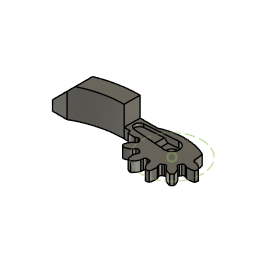
TRGRIP01_Grip_Right_50x15 (Autodesk Fusion 360 design; units mm, degrees)
description: Spur Gear; Module: 2.5; Num Teeth: 12; Pressure Angle: 20.0; Backlash: 0.00 mm
Autodesk Fusion 360 part; units mm, degrees
sketch "스케치1" plane through (0, 0, 0) normal (0, 0, 1) x (1, 0, 0) in component "Spur Gear (12 teeth)"
  circle A0 centre (0, 0) radius 11.9492
  circle A1 centre (0, 0) radius 2.5
sketch "스케치2" plane through (0, 0, 0) normal (0, 0, 1) x (1, 0, 0) in component "Spur Gear (12 teeth)"
  spline S0 degree 5 poles (13.9458, -2.0479) (13.9559, -2.0494) (13.9759, -2.052) (14.0061, -2.0549) (14.0465, -2.057) (14.0972, -2.0572) (14.1481, -2.0556) (14.199, -2.0528) (14.2501, -2.0495) (14.3011, -2.0457) (14.3522, -2.0415) (14.4034, -2.0367) (14.4546, -2.0311) (14.5058, -2.0247) (14.5571, -2.0173) (14.6084, -2.0091) (14.6597, -2.0003) (14.7111, -1.9908) (14.7624, -1.9808) (14.8137, -1.9703) (14.8651, -1.9594) (14.9164, -1.9479) (14.9678, -1.9358) (15.0191, -1.9232) (15.0705, -1.91) (15.1218, -1.8963) (15.1731, -1.882) (15.2244, -1.8673) (15.2757, -1.8521) (15.3269, -1.8365) (15.3781, -1.8204) (15.4293, -1.8038) (15.4805, -1.7868) (15.5316, -1.7693) (15.5827, -1.7513) (15.6338, -1.7329) (15.6848, -1.7141) (15.7358, -1.6948) (15.7868, -1.6751) (15.8377, -1.655) (15.8886, -1.6345) (15.9394, -1.6136) (15.9902, -1.5922) (16.0409, -1.5705) (16.0916, -1.5483) (16.1422, -1.5258) (16.1928, -1.5028) (16.2433, -1.4794) (16.2937, -1.4557) (16.3441, -1.4316) (16.3944, -1.4071) (16.4447, -1.3822) (16.4949, -1.3569) (16.545, -1.3313) (16.5951, -1.3053) (16.6451, -1.2789) (16.695, -1.2521) (16.7448, -1.225) (16.7946, -1.1975) (16.8443, -1.1697) (16.8939, -1.1415) (16.9435, -1.1129) (16.9929, -1.084) (17.0423, -1.0548) (17.0916, -1.0251) (17.1408, -0.9952) (17.1899, -0.9649) (17.239, -0.9343) (17.2879, -0.9033) (17.3368, -0.8719) (17.3856, -0.8403) (17.4245, -0.8147) (17.4537, -0.7953) (17.4731, -0.7824) (17.4828, -0.7759) knots 0 0 0 0 0 0 0.01428571 0.02857143 0.04285714 0.05714286 0.07142857 0.08571429 0.1 0.11428571 0.12857143 0.14285714 0.15714286 0.17142857 0.18571429 0.2 0.21428571 0.22857143 0.24285714 0.25714286 0.27142857 0.28571429 0.3 0.31428571 0.32857143 0.34285714 0.35714286 0.37142857 0.38571429 0.4 0.41428571 0.42857143 0.44285714 0.45714286 0.47142857 0.48571429 0.5 0.51428571 0.52857143 0.54285714 0.55714286 0.57142857 0.58571429 0.6 0.61428571 0.62857143 0.64285714 0.65714286 0.67142857 0.68571429 0.7 0.71428571 0.72857143 0.74285714 0.75714286 0.77142857 0.78571429 0.8 0.81428571 0.82857143 0.84285714 0.85714286 0.87142857 0.88571429 0.9 0.91428571 0.92857143 0.94285714 0.95714286 0.97142857 0.98571429 1 1 1 1 1 1
  spline S1 degree 5 poles (13.9458, 2.0479) (13.9559, 2.0494) (13.9759, 2.052) (14.0061, 2.0549) (14.0465, 2.057) (14.0972, 2.0572) (14.1481, 2.0556) (14.199, 2.0528) (14.2501, 2.0495) (14.3011, 2.0457) (14.3522, 2.0415) (14.4034, 2.0367) (14.4546, 2.0311) (14.5058, 2.0247) (14.5571, 2.0173) (14.6084, 2.0091) (14.6597, 2.0003) (14.7111, 1.9908) (14.7624, 1.9808) (14.8137, 1.9703) (14.8651, 1.9594) (14.9164, 1.9479) (14.9678, 1.9358) (15.0191, 1.9232) (15.0705, 1.91) (15.1218, 1.8963) (15.1731, 1.882) (15.2244, 1.8673) (15.2757, 1.8521) (15.3269, 1.8365) (15.3781, 1.8204) (15.4293, 1.8038) (15.4805, 1.7868) (15.5316, 1.7693) (15.5827, 1.7513) (15.6338, 1.7329) (15.6848, 1.7141) (15.7358, 1.6948) (15.7868, 1.6751) (15.8377, 1.655) (15.8886, 1.6345) (15.9394, 1.6136) (15.9902, 1.5922) (16.0409, 1.5705) (16.0916, 1.5483) (16.1422, 1.5258) (16.1928, 1.5028) (16.2433, 1.4794) (16.2937, 1.4557) (16.3441, 1.4316) (16.3944, 1.4071) (16.4447, 1.3822) (16.4949, 1.3569) (16.545, 1.3313) (16.5951, 1.3053) (16.6451, 1.2789) (16.695, 1.2521) (16.7448, 1.225) (16.7946, 1.1975) (16.8443, 1.1697) (16.8939, 1.1415) (16.9435, 1.1129) (16.9929, 1.084) (17.0423, 1.0548) (17.0916, 1.0251) (17.1408, 0.9952) (17.1899, 0.9649) (17.239, 0.9343) (17.2879, 0.9033) (17.3368, 0.8719) (17.3856, 0.8403) (17.4245, 0.8147) (17.4537, 0.7953) (17.4731, 0.7824) (17.4828, 0.7759) knots 0 0 0 0 0 0 0.01428571 0.02857143 0.04285714 0.05714286 0.07142857 0.08571429 0.1 0.11428571 0.12857143 0.14285714 0.15714286 0.17142857 0.18571429 0.2 0.21428571 0.22857143 0.24285714 0.25714286 0.27142857 0.28571429 0.3 0.31428571 0.32857143 0.34285714 0.35714286 0.37142857 0.38571429 0.4 0.41428571 0.42857143 0.44285714 0.45714286 0.47142857 0.48571429 0.5 0.51428571 0.52857143 0.54285714 0.55714286 0.57142857 0.58571429 0.6 0.61428571 0.62857143 0.64285714 0.65714286 0.67142857 0.68571429 0.7 0.71428571 0.72857143 0.74285714 0.75714286 0.77142857 0.78571429 0.8 0.81428571 0.82857143 0.84285714 0.85714286 0.87142857 0.88571429 0.9 0.91428571 0.92857143 0.94285714 0.95714286 0.97142857 0.98571429 1 1 1 1 1 1
  arc A0 (17.4828, -0.7759) -> (17.4828, 0.7759) centre (0, 0) ccw
  line L0 (11.8125, -1.7361) -> (13.9458, -2.0479)
  line L1 (11.8125, 1.7361) -> (13.9458, 2.0479)
  line L2 (11.8125, -1.7361) -> (11.8125, 1.7361)
  point P0 (14.1908, -2.0531)
  point P1 (14.4394, -2.0327)
  point P2 (14.6902, -1.9946)
  point P3 (14.9425, -1.9417)
  point P4 (15.196, -1.8754)
  point P5 (15.4504, -1.7967)
  point P6 (15.7053, -1.7063)
  point P7 (15.9604, -1.6047)
  point P8 (16.2156, -1.4922)
  point P9 (16.4704, -1.3692)
  point P10 (16.7248, -1.2358)
  point P11 (16.9785, -1.0924)
  point P12 (17.2312, -0.939)
  point P13 (14.1908, 2.0531)
  point P14 (14.4394, 2.0327)
  point P15 (14.6902, 1.9946)
  point P16 (14.9425, 1.9417)
  point P17 (15.196, 1.8754)
  point P18 (15.4504, 1.7967)
  point P19 (15.7053, 1.7063)
  point P20 (15.9604, 1.6047)
  point P21 (16.2156, 1.4922)
  point P22 (16.4704, 1.3692)
  point P23 (16.7248, 1.2358)
  point P24 (16.9785, 1.0924)
  point P25 (17.2312, 0.939)
sketch "스케치3" plane through (0, 0, 0) normal (0, 0, 1) x (1, 0, 0) in component "Spur Gear (12 teeth)"
sketch "스케치1 (2)" plane through (0, 0, 0) normal (0, 0, 1) x (1, 0, 0) in component "Spur Gear (12 teeth) (1)"
  circle A0 centre (0, 0) radius 11.9492
  circle A1 centre (0, 0) radius 2.5
extrude "돌출1" add sketch "스케치1 (2)" along normal blind 5 in component "Spur Gear (12 teeth) (1)"
sketch "스케치2 (2)" plane through (0, 0, 0) normal (0, 0, 1) x (1, 0, 0) in component "Spur Gear (12 teeth) (1)"
  spline S0 degree 5 poles (13.9458, -2.0479) (13.9559, -2.0494) (13.9759, -2.052) (14.0061, -2.0549) (14.0465, -2.057) (14.0972, -2.0572) (14.1481, -2.0556) (14.199, -2.0528) (14.2501, -2.0495) (14.3011, -2.0457) (14.3522, -2.0415) (14.4034, -2.0367) (14.4546, -2.0311) (14.5058, -2.0247) (14.5571, -2.0173) (14.6084, -2.0091) (14.6597, -2.0003) (14.7111, -1.9908) (14.7624, -1.9808) (14.8137, -1.9703) (14.8651, -1.9594) (14.9164, -1.9479) (14.9678, -1.9358) (15.0191, -1.9232) (15.0705, -1.91) (15.1218, -1.8963) (15.1731, -1.882) (15.2244, -1.8673) (15.2757, -1.8521) (15.3269, -1.8365) (15.3781, -1.8204) (15.4293, -1.8038) (15.4805, -1.7868) (15.5316, -1.7693) (15.5827, -1.7513) (15.6338, -1.7329) (15.6848, -1.7141) (15.7358, -1.6948) (15.7868, -1.6751) (15.8377, -1.655) (15.8886, -1.6345) (15.9394, -1.6136) (15.9902, -1.5922) (16.0409, -1.5705) (16.0916, -1.5483) (16.1422, -1.5258) (16.1928, -1.5028) (16.2433, -1.4794) (16.2937, -1.4557) (16.3441, -1.4316) (16.3944, -1.4071) (16.4447, -1.3822) (16.4949, -1.3569) (16.545, -1.3313) (16.5951, -1.3053) (16.6451, -1.2789) (16.695, -1.2521) (16.7448, -1.225) (16.7946, -1.1975) (16.8443, -1.1697) (16.8939, -1.1415) (16.9435, -1.1129) (16.9929, -1.084) (17.0423, -1.0548) (17.0916, -1.0251) (17.1408, -0.9952) (17.1899, -0.9649) (17.239, -0.9343) (17.2879, -0.9033) (17.3368, -0.8719) (17.3856, -0.8403) (17.4245, -0.8147) (17.4537, -0.7953) (17.4731, -0.7824) (17.4828, -0.7759) knots 0 0 0 0 0 0 0.01428571 0.02857143 0.04285714 0.05714286 0.07142857 0.08571429 0.1 0.11428571 0.12857143 0.14285714 0.15714286 0.17142857 0.18571429 0.2 0.21428571 0.22857143 0.24285714 0.25714286 0.27142857 0.28571429 0.3 0.31428571 0.32857143 0.34285714 0.35714286 0.37142857 0.38571429 0.4 0.41428571 0.42857143 0.44285714 0.45714286 0.47142857 0.48571429 0.5 0.51428571 0.52857143 0.54285714 0.55714286 0.57142857 0.58571429 0.6 0.61428571 0.62857143 0.64285714 0.65714286 0.67142857 0.68571429 0.7 0.71428571 0.72857143 0.74285714 0.75714286 0.77142857 0.78571429 0.8 0.81428571 0.82857143 0.84285714 0.85714286 0.87142857 0.88571429 0.9 0.91428571 0.92857143 0.94285714 0.95714286 0.97142857 0.98571429 1 1 1 1 1 1
  spline S1 degree 5 poles (13.9458, 2.0479) (13.9559, 2.0494) (13.9759, 2.052) (14.0061, 2.0549) (14.0465, 2.057) (14.0972, 2.0572) (14.1481, 2.0556) (14.199, 2.0528) (14.2501, 2.0495) (14.3011, 2.0457) (14.3522, 2.0415) (14.4034, 2.0367) (14.4546, 2.0311) (14.5058, 2.0247) (14.5571, 2.0173) (14.6084, 2.0091) (14.6597, 2.0003) (14.7111, 1.9908) (14.7624, 1.9808) (14.8137, 1.9703) (14.8651, 1.9594) (14.9164, 1.9479) (14.9678, 1.9358) (15.0191, 1.9232) (15.0705, 1.91) (15.1218, 1.8963) (15.1731, 1.882) (15.2244, 1.8673) (15.2757, 1.8521) (15.3269, 1.8365) (15.3781, 1.8204) (15.4293, 1.8038) (15.4805, 1.7868) (15.5316, 1.7693) (15.5827, 1.7513) (15.6338, 1.7329) (15.6848, 1.7141) (15.7358, 1.6948) (15.7868, 1.6751) (15.8377, 1.655) (15.8886, 1.6345) (15.9394, 1.6136) (15.9902, 1.5922) (16.0409, 1.5705) (16.0916, 1.5483) (16.1422, 1.5258) (16.1928, 1.5028) (16.2433, 1.4794) (16.2937, 1.4557) (16.3441, 1.4316) (16.3944, 1.4071) (16.4447, 1.3822) (16.4949, 1.3569) (16.545, 1.3313) (16.5951, 1.3053) (16.6451, 1.2789) (16.695, 1.2521) (16.7448, 1.225) (16.7946, 1.1975) (16.8443, 1.1697) (16.8939, 1.1415) (16.9435, 1.1129) (16.9929, 1.084) (17.0423, 1.0548) (17.0916, 1.0251) (17.1408, 0.9952) (17.1899, 0.9649) (17.239, 0.9343) (17.2879, 0.9033) (17.3368, 0.8719) (17.3856, 0.8403) (17.4245, 0.8147) (17.4537, 0.7953) (17.4731, 0.7824) (17.4828, 0.7759) knots 0 0 0 0 0 0 0.01428571 0.02857143 0.04285714 0.05714286 0.07142857 0.08571429 0.1 0.11428571 0.12857143 0.14285714 0.15714286 0.17142857 0.18571429 0.2 0.21428571 0.22857143 0.24285714 0.25714286 0.27142857 0.28571429 0.3 0.31428571 0.32857143 0.34285714 0.35714286 0.37142857 0.38571429 0.4 0.41428571 0.42857143 0.44285714 0.45714286 0.47142857 0.48571429 0.5 0.51428571 0.52857143 0.54285714 0.55714286 0.57142857 0.58571429 0.6 0.61428571 0.62857143 0.64285714 0.65714286 0.67142857 0.68571429 0.7 0.71428571 0.72857143 0.74285714 0.75714286 0.77142857 0.78571429 0.8 0.81428571 0.82857143 0.84285714 0.85714286 0.87142857 0.88571429 0.9 0.91428571 0.92857143 0.94285714 0.95714286 0.97142857 0.98571429 1 1 1 1 1 1
  arc A0 (17.4828, -0.7759) -> (17.4828, 0.7759) centre (0, 0) ccw
  line L0 (11.8125, -1.7361) -> (13.9458, -2.0479)
  line L1 (11.8125, 1.7361) -> (13.9458, 2.0479)
  line L2 (11.8125, -1.7361) -> (11.8125, 1.7361)
  point P0 (14.1908, -2.0531)
  point P1 (14.4394, -2.0327)
  point P2 (14.6902, -1.9946)
  point P3 (14.9425, -1.9417)
  point P4 (15.196, -1.8754)
  point P5 (15.4504, -1.7967)
  point P6 (15.7053, -1.7063)
  point P7 (15.9604, -1.6047)
  point P8 (16.2156, -1.4922)
  point P9 (16.4704, -1.3692)
  point P10 (16.7248, -1.2358)
  point P11 (16.9785, -1.0924)
  point P12 (17.2312, -0.939)
  point P13 (14.1908, 2.0531)
  point P14 (14.4394, 2.0327)
  point P15 (14.6902, 1.9946)
  point P16 (14.9425, 1.9417)
  point P17 (15.196, 1.8754)
  point P18 (15.4504, 1.7967)
  point P19 (15.7053, 1.7063)
  point P20 (15.9604, 1.6047)
  point P21 (16.2156, 1.4922)
  point P22 (16.4704, 1.3692)
  point P23 (16.7248, 1.2358)
  point P24 (16.9785, 1.0924)
  point P25 (17.2312, 0.939)
extrude "돌출2" add sketch "스케치2 (2)" along normal blind 5 in component "Spur Gear (12 teeth) (1)"
fillet "필렛1" radius 1 2 edges at (11.8222, -1.7375, 2.5) (11.8222, 1.7375, 2.5) in component "Spur Gear (12 teeth) (1)"
pattern_circular "C-패턴1" count 6 over 150 about axis through (0, 0, 0) along (0, 0, 1) of "돌출2", "필렛1" in component "Spur Gear (12 teeth) (1)"
sketch "스케치3 (2)" plane through (0, 0, 0) normal (0, 0, 1) x (1, 0, 0) in component "Spur Gear (12 teeth) (1)"
  circle A0 centre (0, 0) radius 15 construction
sketch "스케치4" plane through (0, 0, 0) normal (0, 0, 1) x (1, 0, 0)
  line L0 (-10, -4) -> (-50, -4)
  line L1 (-50, -4) -> (-50, 4)
  line L2 (-50, 4) -> (-10, 4)
  line L3 (-10, 4) -> (-10, -4)
  dimension "d35" = 50
  dimension "d36" = 40
  dimension "d37" = 8
  dimension "d38" = 4
  constraint horizontal L0
  constraint vertical L1
  constraint horizontal L2
  constraint vertical L3
  measures "d35" distance of L1 origin
  measures "d36" distance of L1.end L2.end
  measures "d37" distance of L0.end L1.end
  measures "d38" vertical distance of L1.end origin
extrude "돌출5" add sketch "스케치4" along normal blind 15 sketch seen with x (-0.965926, 0.258819, 0) y (-0.258819, -0.965926, 0) z (0, 0, 1) at (0, 0, 0) in component "Spur Gear (12 teeth) (1)"
extrude "돌출7" cut 1 faces at (9.3142, -3.8761, 8.3333) along direction (0.965926, -0.258819, 0) blind 10 in component "Spur Gear (12 teeth) (1)"
sketch "스케치10" plane through (0, -4, 0) normal (0, -1, 0) x (1, 0, 0)
  line L0 (-50, 15) -> (-20, 15)
  line L1 (-20, 15) -> (-20, 0)
  line L2 (-20, 0) -> (-50, 0)
  line L3 (-50, 0) -> (-50, 15)
  line L4 (-17.0367, 0) -> (-50, 0)
  point P0 (-50, 15)
  constraint horizontal L0
  constraint vertical L1
  constraint horizontal L2
  constraint vertical L3
  constraint coincident L1.end L4
  constraint coincident P0 L0.start
extrude "돌출13" add sketch "스케치10" along normal blind 6 sketch seen with x (-0.965926, 0.258819, 0) y (-0.258819, -0.965926, 0) z (0, 0, 1) at (0, 0, 0) in component "Spur Gear (12 teeth) (1)"
chamfer "챔퍼4" distance 10 angle 45 2 edges at (48.2963, -12.941, 15) (50.108, -6.1795, 15) in component "Spur Gear (12 teeth) (1)"
sketch "스케치6" plane through (0, 0, 5) normal (0, 0, 1) x (-1, 0, 0)
  line L0 (16.5902, -2.3924) -> (0.2933, -3.6884)
  line L1 (16.5902, 2.3924) -> (0.2933, 3.6884)
  arc A0 (16.5902, -2.3924) -> (16.5902, 2.3924) centre (16.4, 0) ccw
  arc A1 (0.2933, 3.6884) -> (0.2933, -3.6884) centre (0, 0) ccw
  line L2 (5.3, -3.2902) -> (5.3, 3.2902)
  dimension "d48" = 7.4
  dimension "d49" = 4.8
  dimension "d50" = 16.4
  dimension "d51" = 5.3
  constraint coincident A1.centre origin
  constraint coincident L1.end A1
  constraint tangent L0 A0
  constraint tangent L0 A1
  constraint equal L0 L1
  constraint coincident L1 A1.start
  constraint horizontal A1.centre A0.centre
  constraint tangent L1 A0
  constraint tangent L1 A1
  constraint coincident L0 L2.start
  constraint coincident L1 L2.end
  constraint vertical L2
  measures "d48" diameter of A1
  measures "d49" diameter of A0
  measures "d50" distance of A1.centre A0.centre
  measures "d51" distance of A1.centre L2
extrude "돌출8" cut sketch "스케치6" against normal blind 1.6 contours L0 L1 A0 L2 sketch seen with x (-0.965926, 0.258819, 0) y (-0.258819, -0.965926, 0) z (0, 0, 1) at (0, 0, 0) in component "Spur Gear (12 teeth) (1)"
extrude "돌출9" cut sketch "스케치6" against normal blind 3.2 contours L0 L1 A1 L2 sketch seen with x (-0.965926, 0.258819, 0) y (-0.258819, -0.965926, 0) z (0, 0, 1) at (0, 0, 0) in component "Spur Gear (12 teeth) (1)"
chamfer "챔퍼3" distance 1.6 angle 45 1 edges at (5.1194, -1.3717, 3.4) in component "Spur Gear (12 teeth) (1)"
sketch "스케치11" plane through (0, 0, 5) normal (0, 0, 1) x (-1, 0, 0)
  circle A0 centre (0, 20) radius 26.5101
  arc A1 (-11.9403, 0.4615) -> (11.2598, -4) centre (0, 0) ccw
  point P0 (11.2598, -4)
  dimension "d70" = 20
  constraint vertical A1.centre A0.centre
  constraint coincident A0 P0
  measures "d70" distance of A1.centre A0.centre
extrude "돌출14" cut sketch "스케치11" against normal blind 5 contours A0 A1 sketch seen with x (-0.965926, 0.258819, 0) y (-0.258819, -0.965926, 0) z (0, 0, 1) at (0, 0, 0) in component "Spur Gear (12 teeth) (1)"
sketch "스케치12" plane through (0, 0, 0) normal (0, 0, -1) x (1, 0, 0)
  circle A0 centre (-20, 50) radius 46
  circle A1 centre (-20, 50) radius 54
  line L0 (-50, -4) -> (-11.2598, -4)
  line L1 (-50, -4) -> (-20, -4)
  line L2 (-50, -4) -> (-50, 5.1001)
  line L3 (-20, 10) -> (-20, 4)
  line L4 (-20, 10) -> (-42.7156, 10)
  point P0 (-20, 4)
  point P1 (-50, -4)
  point P2 (-20, -4)
  point P3 (-20, 10)
  point P4 (-20, 10)
  dimension "d75" = 50
  dimension "d76" = 20
  constraint concentric A0 A1
  constraint coincident A0 P0
  constraint coincident P1 L0.start
  constraint coincident P2 L1.end
  constraint coincident A1 P2
  constraint coincident A1 L2.end
  constraint coincident P4 P3
  constraint coincident P0 L3.end
  constraint coincident A0 L4.end
  constraint perpendicular L3 L4
  measures "d75" vertical distance of A0.centre origin
  measures "d76" horizontal distance of A0.centre origin
extrude "돌출15" cut sketch "스케치12" against normal blind 15 contours A0 L3 L4 | A1 L0 L1 L2 picked at (-21.9743, 6.1276) sketch seen with x (-0.965926, 0.258819, 0) y (-0.258819, -0.965926, 0) z (0, 0, 1) at (0, 0, 0) in component "Spur Gear (12 teeth) (1)"
component "Spur Gear (12 teeth)" placed x (1, 0, 0) y (0, 1, 0) z (0, 0, 1) at (0, 0, 0)
component "Spur Gear (12 teeth) (1)" placed x (-0.965926, -0.258819, 0) y (0.258819, -0.965926, 0) z (0, 0, 1) at (0, 0, 0)
